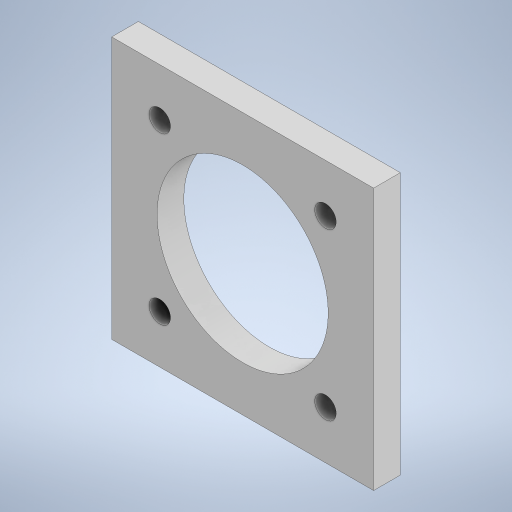
# Autodesk Inventor part: depth-camera
Saved by Autodesk Inventor 2023 (Build 270158000, 158)
## iProperties
Created: 2024-04-08
Part Number: depth-camera
Material: Genérico
Document SubType Name: Modeling
Designer: inigo
Density: 1 g/cm^3
Appearance: Valor por defecto
Author: inigo
Autodesk Inventor part; units mm, degrees
ref_plane "YZ Plane" through (0, 0, 0) normal (1, 0, 0) x (0, 1, 0)
ref_plane "XZ Plane" through (0, 0, 0) normal (0, 1, 0) x (-1, 0, 0)
ref_plane "XY Plane" through (0, 0, 0) normal (0, 0, 1) x (1, 0, 0)
sketch "Boceto1" plane through (0, 0, 0) normal (0, 0, 1) x (1, 0, 0)
  line L0 (-24.5, 24.5) -> (24.5, 24.5)
  line L1 (24.5, 24.5) -> (24.5, -24.5)
  line L2 (24.5, -24.5) -> (-24.5, -24.5)
  line L3 (-24.5, -24.5) -> (-24.5, 24.5)
  line L4 (-24.5, 24.5) -> (24.5, -24.5) construction
  line L5 (24.5, 24.5) -> (-24.5, -24.5) construction
  circle A0 centre (15.5, 15.5) radius 2
  circle A1 centre (-15.5, 15.5) radius 2
  circle A2 centre (-15.5, -15.5) radius 2
  circle A3 centre (15.5, -15.5) radius 2
  circle A4 centre (0, 0) radius 16
  dimension "d0" = 49
  dimension "d1" = 49
  dimension "d2" = 4
  dimension "d3" = 9
  dimension "d6" = 360
  dimension "d10" = 32
  constraints: 12 end point, 5 centre point, 2 midpoint, 2 parallel, 1 coincident, 1 horizontal, 1 perpendicular, 1 point on line, 9 other
  measures "d0" distance of L1.end L2.end
  measures "d1" distance of L0.end L1.end
  measures "d2" diameter of A0
  measures "d3" distance from line of L1 A0.centre
  measures "d10" diameter of A4
extrude "Extrusión1" add sketch "Boceto1" along normal blind 5
